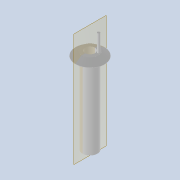
# Autodesk Inventor part: Button
Saved by Autodesk Inventor 2021 (Build 250183000, 183)
## iProperties
Created: 2020-07-21
Part Number: Button
Material: Generic
Document SubType Name: Modeling
Designer: brook
Density: 1 g/cm^3
Appearance: Default
Mass: 1.98339 g
Surface Area: 26.2845 cm^2
Volume: 1.98339 cm^3
Author: brook
Autodesk Inventor part; units mm, degrees
ref_plane "YZ Plane" through (0, 0, 0) normal (1, 0, 0) x (0, 1, 0)
ref_plane "XZ Plane" through (0, 0, 0) normal (0, 1, 0) x (-1, 0, 0)
ref_plane "XY Plane" through (0, 0, 0) normal (0, 0, 1) x (1, 0, 0)
sketch "Sketch1" plane through (0, 0, 0) normal (1, 0, 0) x (0, 1, 0)
  line L0 (0, 4.3419) -> (0, 2.8419)
  line L1 (0, 2.8419) -> (50, 2.8419)
  line L2 (50, 2.8419) -> (50, 5)
  line L3 (50, 5) -> (47, 9)
  line L4 (-10, 0) -> (60, 0) projected
  line L5 (0, 4.3419) -> (47, 4.3419)
  line L6 (47, 4.3419) -> (47, 9)
  point P0 (0, 0)
  dimension "d0" = 5
  dimension "d1" = 50
  dimension "d2" = 0
  dimension "d3" = 9
  dimension "d5" = 3
  constraints: 12 end point, 3 perpendicular, 1 parallel, 1 vertical
  measures "d0" vertical distance of point (0, 0) L2.end
  measures "d1" distance of L0.end L1.end
  measures "d2" distance from line of point (0, 0) L0
  measures "d3" vertical distance of point (0, 0) L3.end
  measures "d5" horizontal distance of L3.end L2.end
revolve "Revolution1" add sketch "Sketch1" angle 360 about axis through (0, -10, 0) along (0, 1, 0)
fillet "Fillet1" radius 0.25 2 edges at (0, 50, -5) (0, 47, -9)
body "Solid1"
